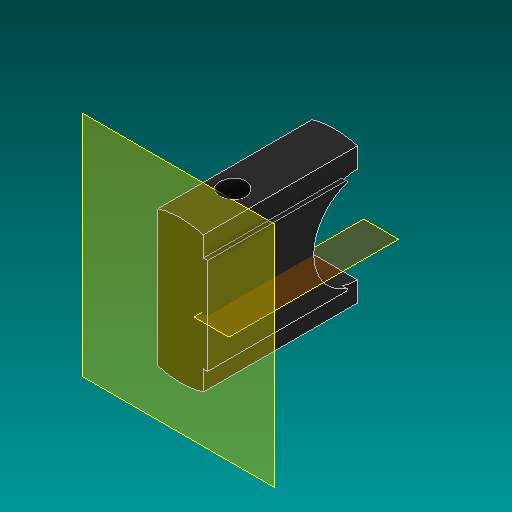
# Autodesk Inventor part: insertLager
Saved by Autodesk Inventor 2020.3 (Build 243373000, 373)
## iProperties
Created: 2020-05-25
Part Number: insertLager
Material: Generic
Document SubType Name: Modeling
Designer: Svend
Density: 1 g/cm^3
Appearance: Default
Author: Svend
Autodesk Inventor part; units mm, degrees
ref_plane "YZ Plane" through (0, 0, 0) normal (1, 0, 0) x (0, 1, 0)
ref_plane "XZ Plane" through (0, 0, 0) normal (0, 1, 0) x (-1, 0, 0)
ref_plane "XY Plane" through (0, 0, 0) normal (0, 0, 1) x (1, 0, 0)
ref_plane "Work Plane1" through (0, 0, 0) normal (0, 0, 1) x (1, 0, 0)
sketch "Sketch1" plane through (0, 0, 0) normal (0, 0, 1) x (1, 0, 0)
  line L0 (-7.7, -28.2497) -> (-11.7, -28.2497) projected
  line L1 (-11.7, -28.2497) -> (-11.7, -31.3497) projected
  arc A0 (-18.7, -31.3497) -> (-11.7, -31.3497) centre (-15.2, -19.3497) ccw projected
  line L2 (-18.7, -31.3497) -> (-18.7, -10.3497) projected
  arc A1 (-11.7, -10.3497) -> (-18.7, -10.3497) centre (-15.2, -22.3497) ccw projected
  line L3 (-11.7, -10.3497) -> (-11.7, -13.4497) projected
  line L4 (-11.7, -13.4497) -> (-7.7, -13.4497) projected
  line L5 (-2, -37) -> (-28.6865, -37) projected
  line L6 (-2, -5) -> (-2, -37) projected
  line L7 (-28.9281, -5) -> (-2, -5) projected
  line L8 (-28.9281, -30) -> (-28.9281, -5) projected
  line L9 (-28.9281, -30) -> (-28.6865, -30) projected
  line L10 (-28.6865, -30) -> (-28.6865, -37) projected
  line L11 (-11.0302, -16.8497) -> (-11.0302, -24.8497) projected
  line L12 (-11.0302, -28.2497) -> (-11.0302, -13.4497)
  line L13 (-7.7, -13.4497) -> (-7.7, -28.2497) projected
  point P0 (0, 0)
  constraints: 2 end point, 2 point on line, 1 collinear, 1 perpendicular, 1 other
extrude "Extrusion1" add sketch "Sketch1" against normal blind 23.787 contours L0 L1 A0 L2 A1 L3 L4 L12 L11
ref_plane "Work Plane2" through (-11.7, -20.8497, 0) normal (0, -1, 0) x (1, 0, 0)
sketch "Sketch2" plane through (-11.7, -20.8497, 0) normal (0, -1, 0) x (1, 0, 0)
  arc A0 (-10.3302, -34.2873) -> (0, -34.2873) centre (-3.5, -22.2873) ccw
  arc A1 (0, -13.2873) -> (-10.3302, -13.2873) centre (-3.5, -25.2873) ccw
  line L0 (0.6698, -23.7873) -> (-10.3302, -23.7873)
  line L1 (0.6698, -29.6873) -> (0, -29.6873)
  line L2 (-10.3302, -23.7873) -> (-10.3302, -34.2873)
  line L3 (0.6698, -23.7873) -> (0.6698, -29.6873)
  line L4 (0, -34.2873) -> (0, -29.6873)
  line L5 (-10.3302, -19.6873) -> (-10.3302, -27.8873) projected
  line L6 (-10.3302, -13.2873) -> (-10.3302, -34.2873) projected
  line L7 (-3.3302, -13.3873) -> (-3.3302, -34.1873) projected
  line L8 (0.6698, -19.7873) -> (0.6698, -27.7873) projected
  line L9 (0.6698, -17.8873) -> (0.6698, -29.6873) projected
  point P0 (11.7, 0)
  point P1 (0, -29.6873)
  point P2 (-3.3302, -23.7873)
  point P3 (0, -29.6873)
  constraints: 10 end point, 2 collinear, 2 midpoint, 1 parallel, 1 perpendicular, 15 other
revolve "Revolution1" [suppressed]
sketch "Sketch3" plane through (-11.7, -20.8497, 0) normal (0, -1, 0) x (1, 0, 0)
  line L0 (-7, 0) -> (-7, -23.787) projected
  line L1 (0, 0) -> (-7, 0) projected
  line L2 (0, 0) -> (0, -23.787) projected
  line L3 (0, 0) -> (0, -23.787) projected
  line L4 (0.6698, 0) -> (0, 0) projected
  line L5 (0.6698, 0) -> (0.6698, -23.787) projected
  circle A0 centre (-3.5, -8) radius 2
  line L6 (0, -23.787) -> (0.6698, -23.787) projected
  line L7 (-7, -23.787) -> (0, -23.787) projected
  point P0 (11.7, 0)
  point P1 (0, -9.3229)
  point P2 (0, -6.6771)
  dimension "d6" = 8
  dimension "d7" = 4
  dimension "d10" = 3.5
  constraints: 1 centre point, 1 coincident
  measures "d6" distance from line of L1 point (-3.5, -8)
  measures "d7" diameter of A0
  measures "d10" distance from line of L0 A0.centre
extrude "Extrusion2" cut sketch "Sketch3" along normal through all both and the other way through all contours A0
sketch "Sketch4" plane through (-11.0302, -28.2497, 0) normal (1, 0, 0) x (0, 0, -1)
  circle A0 centre (23.7873, 7.4) radius 7.4 projected
  point P0 (0, 28.2497)
extrude "Extrusion3" cut sketch "Sketch4" against normal through all
fillet "Fillet2" radius 0.2 2 edges at (-11.3651, -28.2497, -23.787) (-11.3651, -13.4497, -23.787)
body "Solid1"
